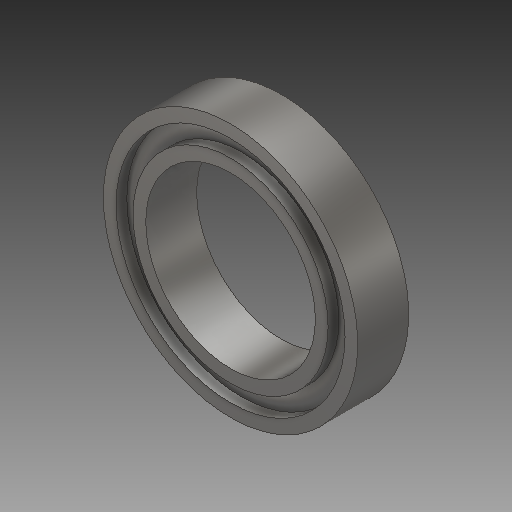
# Autodesk Inventor part: ベアリング10.15
Saved by Autodesk Inventor 2017.3 (Build 213256000, 256)
## iProperties
Part Number: ベアリング10.15
Material: ステンレス鋼
Document SubType Name: Modeling
Designer: 原知也
Density: 8 g/cm^3
Appearance: 半つや出し
Mass: 2.01477 g
Surface Area: 5.3526 cm^2
Volume: 0.251847 cm^3
Author: 原知也
Autodesk Inventor part; units mm, degrees
ref_plane "YZ Plane" through (0, 0, 0) normal (1, 0, 0) x (0, 1, 0)
ref_plane "XZ Plane" through (0, 0, 0) normal (0, 1, 0) x (-1, 0, 0)
ref_plane "XY Plane" through (0, 0, 0) normal (0, 0, 1) x (1, 0, 0)
sketch "スケッチ1" plane through (0, 0, 0) normal (0, 1, 0) x (-1, 0, 0)
  line L0 (0, 0) -> (0, -112.7681) construction
  line L1 (0, -112.7681) -> (0, 117.0869) construction
  line L2 (0, -1.5) -> (5, -1.5) construction
  line L3 (5, -1.5) -> (5, 1.5)
  line L4 (0, 1.5) -> (5, 1.5) construction
  line L5 (7.5, -1.5) -> (7.5, 1.5)
  line L6 (7.5, -1.5) -> (5, 1.5) construction
  line L7 (5, -1.5) -> (7.5, 1.5) construction
  line L8 (7.116, -1.5) -> (5.384, 1.5) construction
  line L9 (5.384, -1.5) -> (7.116, 1.5) construction
  line L10 (6.25, 0) -> (6.25, 1.5) construction
  line L11 (6.75, -0.866) -> (6.75, -1.5)
  line L12 (5.75, -0.866) -> (5.75, -1.5)
  line L13 (6.75, 0.866) -> (6.75, 1.5)
  line L14 (5.75, 0.866) -> (5.75, 1.5)
  line L15 (5, 1.5) -> (5.75, 1.5)
  line L16 (6.75, 1.5) -> (7.5, 1.5)
  arc A0 (6.75, 0.866) -> (5.75, 0.866) centre (6.25, 0) ccw
  arc A1 (5.75, 0.866) -> (5.75, -0.866) centre (6.25, 0) ccw
  arc A2 (5.75, -0.866) -> (6.8902, -0.7682) centre (6.25, 0) ccw
  arc A3 (6.8902, -0.7682) -> (6.75, 0.866) centre (6.25, 0) ccw
  line L17 (5, -1.5) -> (5.75, -1.5)
  line L18 (6.75, -1.5) -> (7.5, -1.5)
  point P0 (6.25, 0)
  dimension "d0" = 5
  dimension "d1" = 1.5
  dimension "d2" = 1.5
  dimension "d3" = 7.5
  dimension "d6" = 30
  dimension "d7" = 30
  dimension "d11" = 1
  constraints: 38 end point, 12 point on line, 9 point on circle, 7 vertical, 5 midpoint, 5 parallel, 4 centre point, 2 horizontal, 2 perpendicular
  measures "d0" distance of L2.start L2.end
  measures "d1" distance of L2.start L0.start
  measures "d2" distance of L0.start L4.start
  measures "d3" distance between parallel lines of L0 L5
  measures "d6" angle of L9 L10
  measures "d7" angle of L10 L8
  measures "d11" radius of A0
revolve "回転2" add sketch "スケッチ1" angle 360 about axis through (0, 0, 0) along (0, 0, -1)
